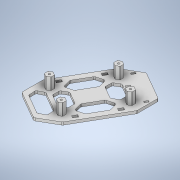
# Autodesk Inventor part: top_body
Saved by Autodesk Inventor 2022 (Build 260153000, 153)
## iProperties
Created: 2022-01-21
Part Number: top_body
Material: Generic
Document SubType Name: Modeling
Designer: felix
Density: 1 g/cm^3
Appearance: Default
Author: felix
Autodesk Inventor part; units mm, degrees
ref_plane "YZ Plane" through (0, 0, 0) normal (1, 0, 0) x (0, 1, 0)
ref_plane "XZ Plane" through (0, 0, 0) normal (0, 1, 0) x (-1, 0, 0)
ref_plane "XY Plane" through (0, 0, 0) normal (0, 0, 1) x (1, 0, 0)
sketch "Sketch1" plane through (0, 0, 0) normal (0, 1, 0) x (-1, 0, 0)
  line L0 (-6.75, 41.2873) -> (6.75, 41.2873)
  line L1 (-8.75, 41.2873) -> (-12.4413, 41.2873)
  line L2 (10.8502, 42.2873) -> (27.4515, 71.0416)
  line L3 (39.1375, 45.1251) -> (-87.6725, 118.3389) construction
  line L4 (27.4515, 73.0416) -> (16.6718, 91.7126)
  line L5 (-8.2867, 49.4115) -> (11.7133, 84.0525) construction
  line L6 (11.7133, 84.0525) -> (-40.2482, 114.0525) construction
  line L7 (-40.2482, 114.0525) -> (-60.2482, 79.4115) construction
  line L8 (-60.2482, 79.4115) -> (-8.2867, 49.4115) construction
  line L9 (27.4515, 73.0416) -> (16.6718, 91.7126)
  line L10 (-13.4413, 41.5553) -> (-38.958, 56.2873)
  line L11 (15.9397, 92.4447) -> (-9.577, 107.1767)
  line L12 (-38.958, 56.2873) -> (-9.577, 107.1767) construction
  line L13 (8.75, 41.2873) -> (9.1181, 41.2873)
  line L14 (6.75, 41.2873) -> (8.75, 41.2873)
  line L15 (-6.75, 41.2873) -> (-8.75, 41.2873)
  line L16 (-68.0523, 76.6802) -> (-74.8023, 88.3716)
  line L17 (-67.0523, 74.9482) -> (-65.2067, 71.7514)
  line L18 (-75.9864, 92.4224) -> (-59.3949, 121.1597)
  line L19 (-57.6644, 122.1597) -> (-36.0952, 122.1767)
  line L20 (-57.6644, 122.1597) -> (-36.0952, 122.1767)
  line L21 (-64.4746, 71.0194) -> (-38.958, 56.2873)
  line L22 (-35.0936, 121.9088) -> (-9.577, 107.1767)
  line L23 (-75.8023, 90.1036) -> (-75.9864, 90.4224)
  line L24 (-74.8023, 88.3716) -> (-75.8023, 90.1036)
  line L25 (-68.0523, 76.6802) -> (-67.0523, 74.9482)
  line L26 (-41.8469, 122.123) -> (-39.8469, 122.123)
  line L27 (8.3599, 47.7766) -> (2.3862, 47.4299)
  line L28 (0.4832, 48.5286) -> (-2.2034, 53.8753)
  line L29 (-2.1483, 55.7733) -> (9.273, 75.5556)
  line L30 (10.8892, 76.5523) -> (16.8629, 76.899)
  line L31 (18.7658, 75.8003) -> (21.4524, 70.4536)
  line L32 (21.3974, 68.5556) -> (9.976, 48.7733)
  line L33 (-53.4825, 79.9302) -> (-55.2145, 76.9302)
  line L34 (-55.6475, 76.6802) -> (-59.1116, 76.6802)
  line L35 (-59.5446, 76.9302) -> (-61.2767, 79.9302)
  line L36 (-61.2767, 80.4302) -> (-59.5446, 83.4302)
  line L37 (-59.1116, 83.6802) -> (-55.6475, 83.6802)
  line L38 (-55.2145, 83.4302) -> (-53.4825, 80.4302)
  circle A0 centre (-57.3796, 80.1802) radius 1.1
  line L39 (-37.3145, 107.9339) -> (-35.5825, 110.9339)
  line L40 (-35.5825, 111.4339) -> (-37.3145, 114.4339)
  line L41 (-37.7475, 114.6839) -> (-41.2116, 114.6839)
  line L42 (-41.6446, 114.4339) -> (-43.3767, 111.4339)
  line L43 (-43.3767, 110.9339) -> (-41.6446, 107.9339)
  line L44 (-41.2116, 107.6839) -> (-37.7475, 107.6839)
  circle A1 centre (-39.4796, 111.1839) radius 1.1
  line L45 (-11.2204, 55.5302) -> (-12.9525, 52.5302)
  line L46 (-12.9525, 52.0302) -> (-11.2204, 49.0302)
  line L47 (-10.7874, 48.7802) -> (-7.3233, 48.7802)
  line L48 (-6.8903, 49.0302) -> (-5.1582, 52.0302)
  line L49 (-5.1582, 52.5302) -> (-6.8903, 55.5302)
  line L50 (-7.3233, 55.7802) -> (-10.7874, 55.7802)
  circle A2 centre (-9.0553, 52.2802) radius 1.1
  line L51 (11.0097, 86.5339) -> (12.7418, 83.5339)
  line L52 (7.1126, 86.7839) -> (10.5767, 86.7839)
  line L53 (4.9475, 83.5339) -> (6.6796, 86.5339)
  circle A3 centre (8.8447, 83.2839) radius 1.1
  line L54 (12.7418, 83.0339) -> (11.0097, 80.0339)
  line L55 (10.5767, 79.7839) -> (7.1126, 79.7839)
  line L56 (6.6796, 80.0339) -> (4.9475, 83.0339)
  line L57 (-55.454, 69.7153) -> (-53.954, 72.3134)
  line L58 (-53.954, 72.3134) -> (-49.6239, 69.8134)
  line L59 (-49.6239, 69.8134) -> (-51.1239, 67.2153)
  line L60 (-51.1239, 67.2153) -> (-55.454, 69.7153)
  line L61 (-29.454, 114.7487) -> (-30.954, 112.1506)
  line L62 (-30.954, 112.1506) -> (-26.6239, 109.6506)
  line L63 (-26.6239, 109.6506) -> (-25.1239, 112.2487)
  line L64 (-25.1239, 112.2487) -> (-29.454, 114.7487)
  line L65 (-19.0809, 48.7153) -> (-17.5809, 51.3134)
  line L66 (-17.5809, 51.3134) -> (-21.9111, 53.8134)
  line L67 (-21.9111, 53.8134) -> (-23.4111, 51.2153)
  line L68 (-23.4111, 51.2153) -> (-19.0809, 48.7153)
  line L69 (2.5889, 96.2487) -> (6.9191, 93.7487)
  line L70 (1.0889, 93.6506) -> (2.5889, 96.2487)
  line L71 (5.4191, 91.1506) -> (1.0889, 93.6506)
  line L72 (6.9191, 93.7487) -> (5.4191, 91.1506)
  line L73 (-46.6628, 74.1138) -> (-44.8326, 67.2837)
  line L74 (-43.9008, 66.0692) -> (-28.0151, 56.8977)
  line L75 (-26.4975, 56.6979) -> (-19.6674, 58.528)
  line L76 (-18.2532, 60.9775) -> (-20.0833, 67.8076)
  line L77 (-21.0151, 69.022) -> (-36.9008, 78.1936)
  line L78 (-38.4184, 78.3934) -> (-45.2485, 76.5633)
  line L79 (18.1755, 76.9752) -> (1.0736, 47.3537) construction
  line L80 (-47.6182, 61.2873) -> (-30.8593, 90.3146) construction
  line L81 (-30.2977, 51.2873) -> (-13.5388, 80.3146) construction
  line L82 (12.9005, 45.8386) -> (-2.6877, 54.8391) construction
  line L83 (25.3698, 67.436) -> (9.8839, 76.3775) construction
  line L84 (-28.8675, 104.936) -> (-22.0374, 106.7661)
  line L85 (-20.5198, 106.5663) -> (-4.6341, 97.3948)
  line L86 (-3.7023, 96.1804) -> (-1.8722, 89.3502)
  line L87 (-3.2864, 86.9007) -> (-10.1165, 85.0706)
  line L88 (-11.6341, 85.2704) -> (-27.5198, 94.442)
  line L89 (-28.4516, 95.6564) -> (-30.2817, 102.4865)
  line L90 (-18.2372, 112.1767) -> (-34.9961, 83.1494) construction
  line L91 (-0.9167, 102.1767) -> (-17.6756, 73.1494) construction
  line L92 (-57.3796, 80.1802) -> (8.8447, 83.2839) construction
  line L93 (-9.0553, 52.2802) -> (-39.4796, 111.1839) construction
  line L94 (-17.7355, 59.0456) -> (-47.1804, 76.0456) construction
  line L95 (-1.3545, 87.4184) -> (-30.7994, 104.4184) construction
  line L96 (-52.6332, 88.8713) -> (-40.5088, 81.8713) construction
  line L97 (-44.6332, 102.7278) -> (-32.5088, 95.7278) construction
  line L98 (-36.602, 102.6382) -> (-48.54, 81.9609) construction
  line L99 (3.5134, 73.5797) -> (-3.3169, 61.7492)
  line L100 (-5.0713, 60.7493) -> (-10.8079, 60.8133)
  line L101 (-12.5063, 61.7939) -> (-15.43, 66.7299)
  line L102 (-15.4413, 68.7492) -> (-8.6109, 80.5797)
  line L103 (-6.8566, 81.5796) -> (-1.12, 81.5156)
  line L104 (0.5785, 80.535) -> (3.5022, 75.599)
  line L105 (-3.9018, 60.7363) -> (-16.0261, 67.7363) construction
  line L106 (4.0982, 74.5927) -> (-8.0261, 81.5927) construction
  line L107 (0.0051, 81.5031) -> (-11.9329, 60.8258) construction
  arc A4 (-57.6644, 122.1597) -> (-59.3949, 121.1597) centre (-57.6628, 120.1597) ccw
  arc A5 (-75.9864, 92.4224) -> (-75.9864, 90.4224) centre (-74.2543, 91.4224) ccw
  arc A6 (-35.0936, 121.9088) -> (-36.0952, 122.1767) centre (-36.0936, 120.1767) ccw
  arc A7 (16.6718, 91.7126) -> (15.9397, 92.4447) centre (14.9397, 90.7126) ccw
  arc A8 (27.4515, 71.0416) -> (27.4515, 73.0416) centre (25.7194, 72.0416) ccw
  arc A9 (9.1181, 41.2873) -> (10.8502, 42.2873) centre (9.1181, 43.2873) ccw
  arc A10 (-13.4413, 41.5553) -> (-12.4413, 41.2873) centre (-12.4413, 43.2873) ccw
  arc A11 (-65.2067, 71.7514) -> (-64.4746, 71.0194) centre (-63.4746, 72.7514) ccw
  arc A12 (-61.2767, 80.4302) -> (-61.2767, 79.9302) centre (-60.8437, 80.1802) ccw
  arc A13 (-59.1116, 83.6802) -> (-59.5446, 83.4302) centre (-59.1116, 83.1802) ccw
  arc A14 (-55.2145, 83.4302) -> (-55.6475, 83.6802) centre (-55.6475, 83.1802) ccw
  arc A15 (-53.4825, 79.9302) -> (-53.4825, 80.4302) centre (-53.9155, 80.1802) ccw
  arc A16 (-55.6475, 76.6802) -> (-55.2145, 76.9302) centre (-55.6475, 77.1802) ccw
  arc A17 (-59.5446, 76.9302) -> (-59.1116, 76.6802) centre (-59.1116, 77.1802) ccw
  arc A18 (-43.3767, 111.4339) -> (-43.3767, 110.9339) centre (-42.9437, 111.1839) ccw
  arc A19 (-41.2116, 114.6839) -> (-41.6446, 114.4339) centre (-41.2116, 114.1839) ccw
  arc A20 (-37.3145, 114.4339) -> (-37.7475, 114.6839) centre (-37.7475, 114.1839) ccw
  arc A21 (-35.5825, 110.9339) -> (-35.5825, 111.4339) centre (-36.0155, 111.1839) ccw
  arc A22 (-37.7475, 107.6839) -> (-37.3145, 107.9339) centre (-37.7475, 108.1839) ccw
  arc A23 (-41.6446, 107.9339) -> (-41.2116, 107.6839) centre (-41.2116, 108.1839) ccw
  arc A24 (7.1126, 86.7839) -> (6.6796, 86.5339) centre (7.1126, 86.2839) ccw
  arc A25 (11.0097, 86.5339) -> (10.5767, 86.7839) centre (10.5767, 86.2839) ccw
  arc A26 (12.7418, 83.0339) -> (12.7418, 83.5339) centre (12.3088, 83.2839) ccw
  arc A27 (10.5767, 79.7839) -> (11.0097, 80.0339) centre (10.5767, 80.2839) ccw
  arc A28 (6.6796, 80.0339) -> (7.1126, 79.7839) centre (7.1126, 80.2839) ccw
  arc A29 (4.9475, 83.5339) -> (4.9475, 83.0339) centre (5.3806, 83.2839) ccw
  arc A30 (-12.9525, 52.5302) -> (-12.9525, 52.0302) centre (-12.5194, 52.2802) ccw
  arc A31 (-11.2204, 49.0302) -> (-10.7874, 48.7802) centre (-10.7874, 49.2802) ccw
  arc A32 (-7.3233, 48.7802) -> (-6.8903, 49.0302) centre (-7.3233, 49.2802) ccw
  arc A33 (-5.1582, 52.0302) -> (-5.1582, 52.5302) centre (-5.5912, 52.2802) ccw
  arc A34 (-6.8903, 55.5302) -> (-7.3233, 55.7802) centre (-7.3233, 55.2802) ccw
  arc A35 (-10.7874, 55.7802) -> (-11.2204, 55.5302) centre (-10.7874, 55.2802) ccw
  arc A36 (-45.2485, 76.5633) -> (-46.6628, 74.1138) centre (-44.7309, 74.6314) ccw
  arc A37 (-36.9008, 78.1936) -> (-38.4184, 78.3934) centre (-37.9008, 76.4616) ccw
  arc A38 (-44.8326, 67.2837) -> (-43.9008, 66.0692) centre (-42.9008, 67.8013) ccw
  arc A39 (-28.0151, 56.8977) -> (-26.4975, 56.6979) centre (-27.0151, 58.6297) ccw
  arc A40 (-19.6674, 58.528) -> (-18.2532, 60.9775) centre (-20.185, 60.4599) ccw
  arc A41 (-20.0833, 67.8076) -> (-21.0151, 69.022) centre (-22.0151, 67.29) ccw
  arc A42 (-28.4516, 95.6564) -> (-27.5198, 94.442) centre (-26.5198, 96.174) ccw
  arc A43 (-28.8675, 104.936) -> (-30.2817, 102.4865) centre (-28.3499, 103.0042) ccw
  arc A44 (-20.5198, 106.5663) -> (-22.0374, 106.7661) centre (-21.5198, 104.8343) ccw
  arc A45 (-3.7023, 96.1804) -> (-4.6341, 97.3948) centre (-5.6341, 95.6627) ccw
  arc A46 (-3.2864, 86.9007) -> (-1.8722, 89.3502) centre (-3.804, 88.8326) ccw
  arc A47 (-11.6341, 85.2704) -> (-10.1165, 85.0706) centre (-10.6341, 87.0025) ccw
  arc A48 (-2.1483, 55.7733) -> (-2.2034, 53.8753) centre (-0.4163, 54.7733) ccw
  arc A49 (10.8892, 76.5523) -> (9.273, 75.5556) centre (11.0051, 74.5556) ccw
  arc A50 (18.7658, 75.8003) -> (16.8629, 76.899) centre (16.9788, 74.9024) ccw
  arc A51 (21.3974, 68.5556) -> (21.4524, 70.4536) centre (19.6653, 69.5556) ccw
  arc A52 (8.3599, 47.7766) -> (9.976, 48.7733) centre (8.244, 49.7733) ccw
  arc A53 (0.4832, 48.5286) -> (2.3862, 47.4299) centre (2.2703, 49.4266) ccw
  arc A54 (-15.4413, 68.7492) -> (-15.43, 66.7299) centre (-13.7092, 67.7492) ccw
  arc A55 (-6.8566, 81.5796) -> (-8.6109, 80.5797) centre (-6.8789, 79.5797) ccw
  arc A56 (0.5785, 80.535) -> (-1.12, 81.5156) centre (-1.1423, 79.5158) ccw
  arc A57 (3.5134, 73.5797) -> (3.5022, 75.599) centre (1.7814, 74.5797) ccw
  arc A58 (-5.0713, 60.7493) -> (-3.3169, 61.7492) centre (-5.049, 62.7492) ccw
  arc A59 (-12.5063, 61.7939) -> (-10.8079, 60.8133) centre (-10.7856, 62.8132) ccw
  line L108 (-45.218, 101.7148) -> (-52.0484, 89.8843)
  line L109 (-52.0371, 87.865) -> (-49.1134, 82.929)
  line L110 (-47.4149, 81.9484) -> (-41.6784, 81.8844)
  line L111 (-37.7271, 102.6507) -> (-43.4636, 102.7147)
  line L112 (-33.1049, 96.7341) -> (-36.0286, 101.6701)
  line L113 (-39.924, 82.8843) -> (-33.0936, 94.7148)
  arc A60 (-41.6784, 81.8844) -> (-39.924, 82.8843) centre (-41.656, 83.8843) ccw
  arc A61 (-33.0936, 94.7148) -> (-33.1049, 96.7341) centre (-34.8257, 95.7148) ccw
  arc A62 (-36.0286, 101.6701) -> (-37.7271, 102.6507) centre (-37.7494, 100.6509) ccw
  arc A63 (-43.4636, 102.7147) -> (-45.218, 101.7148) centre (-43.4859, 100.7148) ccw
  arc A64 (-52.0484, 89.8843) -> (-52.0371, 87.865) centre (-50.3163, 88.8843) ccw
  arc A65 (-49.1134, 82.929) -> (-47.4149, 81.9484) centre (-47.3926, 83.9483) ccw
  point P0 (10.2728, 41.2873)
  point P1 (-12.9772, 41.2873)
  point P2 (28.0288, 72.0416)
  point P3 (19.1508, 56.6645)
  point P4 (-67.6857, 106.7996)
  point P5 (-8.2867, 49.4115)
  point P6 (-24.2675, 81.732)
  point P7 (9.4367, 47.8391)
  point P8 (21.9367, 69.4898)
  point P9 (-53.3381, 80.1802)
  point P10 (-55.3588, 76.6802)
  point P11 (-59.4003, 76.6802)
  point P12 (-61.421, 80.1802)
  point P13 (-59.4003, 83.6802)
  point P14 (-55.3588, 83.6802)
  point P15 (-37.4588, 107.6839)
  point P16 (-35.4381, 111.1839)
  point P17 (-37.4588, 114.6839)
  point P18 (-41.5003, 114.6839)
  point P19 (-43.521, 111.1839)
  point P20 (-41.5003, 107.6839)
  point P21 (-11.0761, 55.7802)
  point P22 (-13.0968, 52.2802)
  point P23 (-11.0761, 48.7802)
  point P24 (-7.0346, 48.7802)
  point P25 (-5.0139, 52.2802)
  point P26 (-7.0346, 55.7802)
  point P27 (10.8654, 86.7839)
  point P28 (12.8861, 83.2839)
  point P29 (6.8239, 86.7839)
  point P30 (4.8032, 83.2839)
  point P31 (10.8654, 79.7839)
  point P32 (6.8239, 79.7839)
  point P33 (-44.6182, 66.4835)
  point P34 (-27.2977, 56.4835)
  point P35 (-20.2977, 68.6078)
  point P36 (-37.6182, 78.6078)
  point P37 (-21.2372, 106.9806)
  point P38 (-3.9167, 96.9806)
  point P39 (-10.9167, 84.8562)
  point P40 (-28.2372, 94.8562)
  point P41 (8.8447, 83.2839)
  dimension "d82" = 23.25
  dimension "d88" = 120
  dimension "d89" = 120
  dimension "d90" = 35.512
  dimension "d91" = 17.756
  dimension "d92" = 17.756
  dimension "d95" = 40
  dimension "d97" = 20
  dimension "d99" = 30
  dimension "d102" = 60
  dimension "d145" = 180
  dimension "d146" = 30
  dimension "d147" = 8.1242
  dimension "d148" = 8.1242
  dimension "d155" = 2.2
  dimension "d156" = 7
  dimension "d157" = 1
  dimension "d158" = 1
  dimension "d160" = 3
  dimension "d162" = 3
  dimension "d163" = 9
  dimension "d169" = 6
  dimension "d170" = 10
  dimension "d171" = 20
  dimension "d172" = 14
  dimension "d179" = 7
  dimension "d181" = 2
  dimension "d186" = 0.5
  dimension "d187" = 0.5
  dimension "d189" = 2
  dimension "d190" = 2
  dimension "d191" = 4
  dimension "d192" = 16
  dimension "d193" = 8
  dimension "d194" = 14
  dimension "d195" = 8
  dimension "d204" = 14
  dimension "d206" = 18.762
  dimension "d207" = 28.2702
  dimension "d238" = 5
  dimension "d244" = 25
  dimension "d245" = 12.5
  dimension "d246" = 0
  dimension "d247" = 4
  constraints: 228 end point, 124 point on circle, 112 tangent, 110 point on line, 79 symmetric about line, 66 centre point, 51 equal radius, 16 parallel, 9 equal length, 6 perpendicular, 4 collinear, 3 coincident, 3 midpoint, 2 horizontal, 22 other
  measures "d82" distance of point (10.273, 41.287) point (-12.977, 41.287)
  measures "d88" angle of L2 L1
  measures "d89" angle of L4 L2
  measures "d90" distance of point (10.273, 41.287) point (28.029, 72.042)
  measures "d91" distance of point (19.151, 56.664) point (10.273, 41.287)
  measures "d92" distance of point (28.029, 72.042) point (19.151, 56.664)
  measures "d95" distance of L5.start L5.end
  measures "d97" distance from line of L3 L5.start
  measures "d99" distance of L10.end point (-12.977, 41.287)
  measures "d102" distance of L7.end L5.start
  measures "d145" angle of L10 L21
  measures "d146" distance from line of L5 point (-24.267, 81.732)
  measures "d147" distance from line of L0 L5.start
  measures "d148" distance from line of L4 L5.end
  measures "d155" diameter of A0
  measures "d156" distance between parallel lines of L38 L35
  measures "d157" distance edge to line of A0 L7
  measures "d158" distance edge to line of A0 L8
  measures "d160" distance between parallel lines of L58 L60
  measures "d162" distance between parallel lines of L8 L58
  measures "d163" distance between parallel lines of L57 L7
  measures "d169" distance between parallel lines of L21 L74
  measures "d170" distance from line of L12 point (-27.298, 56.483)
  measures "d171" distance of point (-44.618, 66.483) point (-27.298, 56.483)
  measures "d172" distance between parallel lines of L77 L74
  measures "d179" distance from line of L94.end L80
  measures "d181" radius of A4
  measures "d186" radius of A12
  measures "d187" radius of A27
  measures "d189" radius of A36
  measures "d190" radius of A54
  measures "d191" distance between parallel lines of L29 L99
  measures "d192" distance of L105.start L106.start
  measures "d193" distance from line of L3 L106.start
  measures "d194" distance between parallel lines of L99 L102
  measures "d195" distance between parallel lines of L106 L3
  measures "d204" distance between parallel lines of L32 L29
  measures "d206" distance between parallel lines of L88 L77
  measures "d207" distance between parallel lines of L113 L102
  measures "d238" distance of L59.end L57.start
  measures "d244" distance of point (21.937, 69.49) point (9.437, 47.839)
  measures "d245" distance from line of L3 point (9.437, 47.839)
  measures "d246" angle of L83 L82
  measures "d247" distance between parallel lines of L2 L32
extrude "Extrusion1_main_body" add sketch "Sketch1" along normal blind 3 contours L15 L1 A10 L10 L21 A11 L17 L25 L16 L24 L23 A5 L18 A4 L19 A6 L22 L11 A7 L4 A8 L2 A9 L13 L14 L0
extrude "Extrusion2_main_body" add sketch "Sketch1" along normal blind 16 contours L33 A16 L34 A17 L35 A12 L36 A13 L37 A14 L38 A15 | A22 L44 A23 L43 A18 L42 A19 L41 A20 L40 A21 L39 | A35 L50 A34 L49 A33 L48 A32 L47 A31 L46 A30 L45 | L51 A26 L54 A27 L55 A28 L56 A29 L53 A24 L52 A25
extrude "Extrusion3_main_body" add sketch "Sketch1" along normal blind 13 contours A0 | A1 | A2 | A3
sketch "Sketch2_insert" plane through (0, 0, 0) normal (0, -1, 0) x (1, 0, 0)
  line L0 (43.6332, 119.4597) -> (66.6332, 79.6225)
  line L1 (66.6332, 79.6225) -> (65.0744, 78.7225)
  line L2 (65.0744, 78.7225) -> (42.0744, 118.5597)
  line L3 (42.0744, 118.5597) -> (43.6332, 119.4597)
  line L4 (59.3949, 121.1597) -> (75.9864, 92.4224) projected
  line L5 (52.0484, 89.8843) -> (45.218, 101.7148) projected
  line L6 (64.4746, 71.0194) -> (13.4413, 41.5553) projected
  line L7 (-15.9397, 92.4447) -> (35.0936, 121.9088) projected
  line L8 (66.7277, 106.2351) -> (52.3982, 97.962) construction
  line L9 (59.3949, 121.1597) -> (75.9864, 92.4224) projected
  line L10 (51.0744, 102.9712) -> (47.3505, 100.8212)
  line L11 (47.3505, 100.8212) -> (52.3505, 92.1609)
  line L12 (52.3505, 92.1609) -> (56.0744, 94.3109)
  line L13 (52.6332, 103.8712) -> (54.6251, 105.0212)
  line L14 (54.6251, 105.0212) -> (59.6251, 96.3609)
  line L15 (59.6251, 96.3609) -> (57.6332, 95.2109)
  line L16 (46.9483, 118.7178) -> (50.4124, 120.7178)
  line L17 (50.4124, 120.7178) -> (51.4124, 118.9857)
  line L18 (51.4124, 118.9857) -> (47.9483, 116.9857)
  line L19 (47.9483, 116.9857) -> (46.9483, 118.7178)
  line L20 (36.0952, 122.1767) -> (57.6644, 122.1597) projected
  line L21 (67.6483, 82.8643) -> (71.1124, 84.8643)
  line L22 (71.1124, 84.8643) -> (70.1124, 86.5964)
  line L23 (70.1124, 86.5964) -> (66.6483, 84.5964)
  line L24 (66.6483, 84.5964) -> (67.6483, 82.8643)
  point P0 (0, 0)
  point P1 (55.1332, 99.5411)
  point P2 (67.6906, 106.7911)
  point P3 (49.8505, 96.4911)
  dimension "d249" = 1.8
  dimension "d251" = 46
  dimension "d252" = 23
  dimension "d254" = 10
  dimension "d255" = 4.3
  dimension "d256" = 1.4
  dimension "d258" = 2.3
  dimension "d265" = 4
  dimension "d266" = 2
  dimension "d267" = 2.5
  dimension "d268" = 2.3
  dimension "d269" = 1.4477
  dimension "d272" = 8
  dimension "d273" = 10
  constraints: 38 end point, 12 parallel, 7 point on line, 6 perpendicular, 4 symmetric about line, 3 midpoint
  measures "d249" distance of L2.end L0.start
  measures "d251" distance of L0.start L0.end
  measures "d252" distance of L0.start point (55.133, 99.541)
  measures "d254" distance between parallel lines of L12 L10
  measures "d255" distance of L11.end L12.end
  measures "d256" distance between parallel lines of L5 L11
  measures "d258" distance of L13.start L13.end
  measures "d265" distance of L16.start L16.end
  measures "d266" distance between parallel lines of L18 L16
  measures "d267" distance between parallel lines of L0 L19
  measures "d268" distance between parallel lines of L16 L3
  measures "d269" distance from line of L16.end L20
  measures "d272" distance between parallel lines of L17 L4
  measures "d273" distance between parallel lines of L15 L13
extrude "Extrusion1_feature1" cut sketch "Sketch2_insert" against normal blind 1.5 contours L0 L1 L2 L3
extrude "Extrusion2_feature1" cut sketch "Sketch2_insert" against normal blind 1.2 contours L13 L14 L15 L0
extrude "Extrusion3_feature1" cut sketch "Sketch2_insert" against normal blind 3 contours L2 L12 L11 L10
extrude "Extrusion4_feature1_zip_ties" cut sketch "Sketch2_insert" against normal blind 3 contours L16 L17 L18 L19 | L24 L23 L22 L21
body "Solid1"
